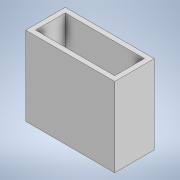
# Autodesk Inventor part: spacer-1x2_250
Saved by Autodesk Inventor 2022.1 (Build 261234000, 234)
## iProperties
Created: 2021-08-08
Part Number: spacer-1x2_250
Material: Generic
Document SubType Name: Modeling
Designer: robst
Density: 1 g/cm^3
Appearance: Default
Author: robst
Autodesk Inventor part; units mm, degrees
ref_plane "YZ Plane" through (0, 0, 0) normal (1, 0, 0) x (0, 1, 0)
ref_plane "XZ Plane" through (0, 0, 0) normal (0, 1, 0) x (-1, 0, 0)
ref_plane "XY Plane" through (0, 0, 0) normal (0, 0, 1) x (1, 0, 0)
sketch "Sketch1" plane through (0, 0, 0) normal (0, 1, 0) x (-1, 0, 0)
  line L0 (-28.575, 12.7) -> (-28.575, -12.7)
  line L1 (-28.575, -12.7) -> (28.575, -12.7)
  line L2 (28.575, -12.7) -> (28.575, 12.7)
  line L3 (28.575, 12.7) -> (-28.575, 12.7)
  line L4 (-28.575, 12.7) -> (28.575, -12.7) construction
  line L5 (-28.575, -12.7) -> (28.575, 12.7) construction
  line L6 (-25.4, 9.525) -> (-25.4, -9.525)
  line L7 (-25.4, -9.525) -> (25.4, -9.525)
  line L8 (25.4, -9.525) -> (25.4, 9.525)
  line L9 (25.4, 9.525) -> (-25.4, 9.525)
  line L10 (-25.4, 9.525) -> (25.4, -9.525) construction
  line L11 (-25.4, -9.525) -> (25.4, 9.525) construction
  point P0 (0, 0)
  dimension "d0" = 25.4
  dimension "d1" = 57.15
  dimension "d2" = 3.175
  dimension "d3" = 3.175
  constraints: 24 end point, 5 parallel, 4 midpoint, 2 perpendicular, 1 vertical
  measures "d0" distance of L1.end L2.end
  measures "d1" distance of L2.end L0.start
  measures "d2" distance between parallel lines of L2 L8
  measures "d3" distance between parallel lines of L1 L7
extrude "Extrusion1" add sketch "Sketch1" along normal blind 50.8
body "Solid1"
